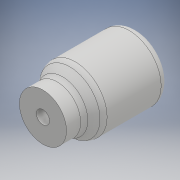
# Autodesk Inventor part: Top Knob
Saved by Autodesk Inventor 2017 (Build 210142000, 142)
## iProperties
Created: 2017-03-04
Part Number: Top Knob
Material: Generic
Document SubType Name: Modeling
Designer: aribu
Density: 1 g/cm^3
Appearance: Default
Author: aribu
Autodesk Inventor part; units mm, degrees
ref_plane "YZ Plane" through (0, 0, 0) normal (1, 0, 0) x (0, 1, 0)
ref_plane "XZ Plane" through (0, 0, 0) normal (0, 1, 0) x (-1, 0, 0)
ref_plane "XY Plane" through (0, 0, 0) normal (0, 0, 1) x (1, 0, 0)
sketch "Sketch2" plane through (0, 0, 0) normal (0, 0, 1) x (1, 0, 0)
  line L0 (4.2, -19.2857) -> (4.2, 20.7143)
  line L1 (4.2, -19.2857) -> (15, -19.2857)
  line L2 (15, -19.2857) -> (15, -8.3281)
  line L3 (15, -8.3281) -> (20.3713, -0.6476)
  line L4 (20.3713, -0.6476) -> (20.3713, 40.7143)
  line L5 (20.3713, 40.7143) -> (0, 40.7143)
  line L6 (0, 40.7143) -> (0, 20.7143)
  line L7 (0, 20.7143) -> (4.2, 20.7143)
  point P0 (0, 0)
  dimension "d3" = 4.2
  dimension "d4" = 10.8
  dimension "d5" = 60
  dimension "d6" = 20
  constraints: 16 end point, 3 vertical, 2 perpendicular, 1 horizontal, 1 parallel
  measures "d3" distance from line of point (0, 0) L0
  measures "d4" distance of L0.start L1.end
  measures "d5" distance between parallel lines of L1 L5
  measures "d6" distance of L5.end L6.end
revolve "Revolution1" add sketch "Sketch2" angle 360 about axis through (0, 40.7143, 0) along (0, -1, 0)
fillet "Fillet1" radius 6 2 edges at (-20.3713, -0.6476, 0) (-15, -8.3281, 0)
fillet "Fillet2" radius 5 1 edges at (-20.3713, 40.7143, 0)
body "Solid1"
